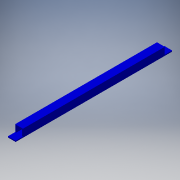
# Autodesk Inventor part: 2018 Top Cross Bar
Saved by Autodesk Inventor 2018 (Build 220112000, 112)
## iProperties
Created: 2018-01-26
Part Number: 2018 Top Cross Bar
Material: Generic
Document SubType Name: Modeling
Designer: Apple
Density: 1 g/cm^3
Appearance: Default
Author: Apple
Autodesk Inventor part; units mm, degrees
ref_plane "YZ Plane" through (0, 0, 0) normal (1, 0, 0) x (0, 1, 0)
ref_plane "XZ Plane" through (0, 0, 0) normal (0, 1, 0) x (-1, 0, 0)
ref_plane "XY Plane" through (0, 0, 0) normal (0, 0, 1) x (1, 0, 0)
sketch "Sketch1" plane through (0, 0, 0) normal (0, 0, 1) x (1, 0, 0)
  line L0 (-305.1624, -66.0045) -> (-279.7624, -66.0045)
  line L1 (-279.7624, -66.0045) -> (-279.7624, -40.6045)
  line L2 (-279.7624, -40.6045) -> (-305.1624, -40.6045)
  line L3 (-305.1624, -40.6045) -> (-305.1624, -66.0045)
  line L4 (-301.9874, -62.8295) -> (-282.9374, -62.8295)
  line L5 (-282.9374, -62.8295) -> (-282.9374, -43.7795)
  line L6 (-282.9374, -43.7795) -> (-301.9874, -43.7795)
  line L7 (-301.9874, -43.7795) -> (-301.9874, -62.8295)
  point P0 (0, 0)
  dimension "d0" = 25.4
  dimension "d1" = 25.4
  dimension "d2" = 3.175
  constraints: 16 end point, 4 parallel, 2 perpendicular, 1 horizontal, 3 other
  measures "d0" distance of L0.start L0.end
  measures "d1" distance of L2.end L0.start
  measures "d2" distance between parallel lines of L3 L7
extrude "Extrusion1" add sketch "Sketch1" along normal blind 508
sketch "Sketch2" plane through (-305.1624, -66.0045, 0) normal (-1, 0, 0) x (0, 0, 1)
  line L0 (508, 3.175) -> (508, 22.225) projected
  line L1 (508, 3.175) -> (484.1875, 3.175)
  line L2 (484.1875, 3.175) -> (484.1875, 25.4)
  line L3 (484.1875, 25.4) -> (508, 25.4)
  line L4 (508, 25.4) -> (508, 3.175)
  line L5 (0, 3.175) -> (0, 22.225) projected
  line L6 (0, 25.4) -> (508, 25.4) projected
  line L7 (0, 3.175) -> (23.8125, 3.175)
  line L8 (23.8125, 3.175) -> (23.8125, 25.4)
  line L9 (23.8125, 25.4) -> (0, 25.4)
  line L10 (0, 25.4) -> (0, 3.175)
  point P0 (0, 66.0045)
  point P1 (496.0938, 25.4)
  dimension "d5" = 460.375
  dimension "d6" = 508
  dimension "d7" = 23.8125
  constraints: 16 end point, 4 parallel, 2 horizontal, 2 perpendicular, 1 horizontal alignment, 1 midpoint, 1 point on line
  measures "d5" distance between parallel lines of L8 L2
  measures "d6" distance between parallel lines of L5 L0
  measures "d7" distance of L5.start L7.end
extrude "Extrusion2" cut sketch "Sketch2" against normal through all
equation "\"d7\" = -0.5 * d5 + 0.5 * d6"
body "Solid1"
